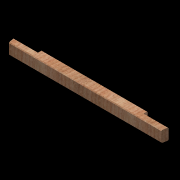
# Autodesk Inventor part: DNW_CON_V2
Saved by Autodesk Inventor 2016 (Build 200138000, 138)
## iProperties
Created: 2017-08-29
Part Number: DNW_CON_V2
Material: Wood (Birch)
Document SubType Name: Modeling
Designer: ludwi
Density: 0.55 g/cm^3
Appearance: Birch - Natural Polished
Author: ludwi
Autodesk Inventor part; units mm, degrees
ref_plane "YZ Plane" through (0, 0, 0) normal (1, 0, 0) x (0, 1, 0)
ref_plane "XZ Plane" through (0, 0, 0) normal (0, 1, 0) x (-1, 0, 0)
ref_plane "XY Plane" through (0, 0, 0) normal (0, 0, 1) x (1, 0, 0)
sketch "Sketch1" plane through (0, 0, 0) normal (0, 0, 1) x (1, 0, 0)
  line L0 (-357.2554, -61.8782) -> (-427.6081, -61.8782) construction
  line L1 (-357.2554, -61.8782) -> (-357.2554, -55.8782) construction
  line L2 (-405.0222, -45.9997) -> (-425.3346, 69.1978) construction
  line L3 (-419.5247, 76.1218) -> (-425.3346, 69.1978) construction
  line L4 (-408.3518, 76.1218) -> (-408.3518, 82.1218) construction
  line L5 (-450.7203, 69.1978) -> (-427.6081, -61.8782) construction
  line L6 (13.9045, -61.8782) -> (-56.4482, -61.8782) construction
  line L7 (13.9045, -61.8782) -> (37.0167, 69.1978) construction
  line L8 (-5.3518, 82.1218) -> (-5.3518, 76.1218) construction
  line L9 (11.631, 69.1978) -> (5.8211, 76.1218) construction
  line L10 (11.631, 69.1978) -> (-8.6814, -45.9997) construction
  line L11 (-56.4482, -55.8782) -> (-56.4482, -61.8782) construction
  line L12 (13.5518, -63.8782) -> (13.9045, -61.8782) construction
  line L13 (13.9045, -61.8782) -> (-56.4482, -61.8782) construction
  line L14 (-56.4482, -61.8782) -> (-56.4482, -63.8782) construction
  line L15 (-56.4482, -63.8782) -> (13.5518, -63.8782) construction
  line L16 (-357.2554, -63.8782) -> (-357.2554, -61.8782) construction
  line L17 (-357.2554, -61.8782) -> (-427.6081, -61.8782) construction
  line L18 (-427.6081, -61.8782) -> (-427.2554, -63.8782) construction
  line L19 (-427.2554, -63.8782) -> (-357.2554, -63.8782) construction
  line L20 (-347.2554, -53.8782) -> (-66.4482, -53.8782)
  line L21 (-56.4482, -63.8782) -> (13.5518, -63.8782)
  line L22 (13.5518, -63.8782) -> (10.3779, -81.8782)
  line L23 (10.3779, -81.8782) -> (-424.0815, -81.8782)
  line L24 (-424.0815, -81.8782) -> (-427.2554, -63.8782)
  line L25 (-427.2554, -63.8782) -> (-357.2554, -63.8782)
  line L26 (45.2684, 76.1218) -> (37.0167, 69.1978) projected
  line L27 (94.6482, 76.1218) -> (94.6482, 82.1218) projected
  line L28 (-508.3518, 82.1218) -> (-508.3518, 76.1218) projected
  line L29 (-450.7203, 69.1978) -> (-458.972, 76.1218) projected
  line L30 (-5.3518, 82.1218) -> (94.6482, 82.1218) projected
  line L31 (-508.3518, 82.1218) -> (-408.3518, 82.1218) projected
  line L32 (-56.4482, -55.8782) -> (-20.4541, -55.8782) projected
  line L33 (94.6482, 76.1218) -> (45.2684, 76.1218) projected
  line L34 (5.8211, 76.1218) -> (-5.3518, 76.1218) projected
  line L35 (-20.4541, -55.8782) -> (-8.6814, -45.9997) projected
  line L36 (-405.0222, -45.9997) -> (-393.2495, -55.8782) projected
  line L37 (-408.3518, 76.1218) -> (-419.5247, 76.1218) projected
  line L38 (-458.972, 76.1218) -> (-508.3518, 76.1218) projected
  line L39 (-393.2495, -55.8782) -> (-357.2554, -55.8782) projected
  line L40 (-66.4482, -53.8782) -> (-56.4482, -53.8782)
  line L41 (-56.4482, -53.8782) -> (-56.4482, -63.8782)
  line L42 (-357.2554, -63.8782) -> (-357.2554, -53.8782)
  line L43 (-357.2554, -53.8782) -> (-347.2554, -53.8782)
  point P0 (0, 0)
  dimension "d0" = 28
  constraints: 20 end point, 4 collinear, 2 horizontal, 2 perpendicular, 1 parallel, 1 point on line
  measures "d0" distance between parallel lines of L20 L23
extrude "Extrusion1" add sketch "Sketch1" against normal blind 32
chamfer "Chamfer1" distance 2 angle 45 8 edges at (-392.2554, -63.8782, 0) (-392.2554, -63.8782, -32) (-206.8518, -81.8782, -32) (-206.8518, -81.8782, 0) (-21.4482, -63.8782, 0) (-21.4482, -63.8782, -32) (-206.8518, -53.8782, 0) (-206.8518, -53.8782, -32)
body "Solid1"
